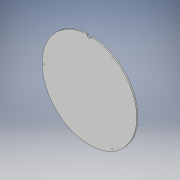
# Autodesk Inventor part: Nap
Saved by Autodesk Inventor 2019 (Build 230136000, 136)
## iProperties
Created: 2021-01-20
Part Number: Nap
Material: Generic
Document SubType Name: Modeling
Designer: Admin
Density: 1 g/cm^3
Appearance: Default
Author: Admin
Autodesk Inventor part; units mm, degrees
ref_plane "YZ Plane" through (0, 0, 0) normal (1, 0, 0) x (0, 1, 0)
ref_plane "XZ Plane" through (0, 0, 0) normal (0, 1, 0) x (-1, 0, 0)
ref_plane "XY Plane" through (0, 0, 0) normal (0, 0, 1) x (1, 0, 0)
sketch "Sketch1" plane through (0, 0, 0) normal (0, 0, 1) x (1, 0, 0)
  arc A0 (-9.9968, 197.2468) -> (9.9968, 197.2468) centre (0, 0) ccw
  arc A1 (-9.9968, 197.2468) -> (9.9968, 197.2468) centre (0, 197.5) ccw
  line L0 (0, 0) -> (197.5, 0) construction
  circle A2 centre (95, 164.5448) radius 1.5
  circle A3 centre (-190, 0) radius 1.5
  circle A4 centre (95, -164.5448) radius 1.5
  dimension "d0" = 395
  dimension "d1" = 20
  dimension "d7" = 3
  dimension "d10" = 360
  constraints: 5 centre point, 5 point on circle, 2 end point, 1 coincident, 1 horizontal, 7 other
  measures "d0" diameter of A0
  measures "d1" diameter of A1
  measures "d7" diameter of A2
extrude "Extrusion1" add sketch "Sketch1" along normal blind 5
body "Solid1"
